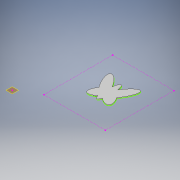
# Autodesk Inventor part: Butterfly
Saved by Autodesk Inventor 2019 (Build 230136000, 136)
## iProperties
Created: 2019-02-04
Part Number: Butterfly
Material: Generic
Document SubType Name: Modeling
Designer: mrhftc
Density: 1 g/cm^3
Appearance: Default
Author: mrhftc
Autodesk Inventor part; units mm, degrees
ref_plane "YZ Plane" through (0, 0, 0) normal (1, 0, 0) x (0, 1, 0)
ref_plane "XZ Plane" through (0, 0, 0) normal (0, 1, 0) x (-1, 0, 0)
ref_plane "XY Plane" through (0, 0, 0) normal (0, 0, 1) x (1, 0, 0)
ref_plane "Work Plane2" through (0, 2.54, 0) normal (0, 1, 0) x (1, 0, 0)
sketch "Sketch5" plane through (0, 2.54, 0) normal (0, 1, 0) x (1, 0, 0)
  ellipse E0 centre (201.451, 177.3473) end of major axis (229.2052, 221.1135) minor radius 16.0156 (208.013, 158.6416) -> (186.5008, 183.6371) ccw
  ellipse E1 centre (187.6899, 154.5313) end of major axis (215.633, 123.3862) minor radius 18.4642 (184.5561, 132.1117) -> (208.013, 158.6416) ccw
  ellipse E2 centre (176.9986, 162.7883) end of major axis (176.9986, 205.3655) minor radius 10.8982 (186.5008, 183.6371) -> (176.9986, 205.3655) ccw
  ellipse E3 centre (176.9986, 162.7883) end of major axis (176.9986, 205.3655) minor radius 10.8982 (176.9986, 120.211) -> (184.5561, 132.1117) ccw
  ellipse E4 centre (152.5463, 177.3473) end of major axis (124.7921, 221.1135) minor radius 16.0156 (167.4964, 183.6371) -> (145.9843, 158.6416) ccw
  ellipse E5 centre (166.3073, 154.5313) end of major axis (138.3642, 123.3862) minor radius 18.4642 (145.9843, 158.6416) -> (169.4411, 132.1117) ccw
  ellipse E6 centre (176.9986, 162.7883) end of major axis (176.9986, 205.3655) minor radius 10.8982 (176.9986, 205.3655) -> (167.4964, 183.6371) ccw
  ellipse E7 centre (176.9986, 162.7883) end of major axis (176.9986, 205.3655) minor radius 10.8982 (169.4411, 132.1117) -> (176.9986, 120.211) ccw
  ellipse E8 centre (166.3073, 154.5313) end of major axis (138.3642, 123.3862) minor radius 18.4642 (145.9843, 158.6416) -> (169.4411, 132.1117) ccw
  ellipse E9 centre (187.6899, 154.5313) end of major axis (215.633, 123.3862) minor radius 18.4642 (184.5561, 132.1117) -> (208.013, 158.6416) ccw
  point P0 (0, 0)
  constraints: 2 coincident, 40 other
ref_plane "Work Plane1" through (0, 2.54, 0) normal (0, 1, 0) x (1, 0, 0)
sketch "Sketch7" plane through (0, 2.54, 0) normal (0, 1, 0) x (1, 0, 0)
  ellipse E0 centre (152.5463, 177.3473) end of major axis (124.7921, 221.1135) minor radius 16.0156 (167.4964, 183.6371) -> (145.9843, 158.6416) ccw construction
  ellipse E1 centre (176.9986, 162.7883) end of major axis (176.9986, 205.3655) minor radius 10.8982 (186.5008, 183.6371) -> (167.4964, 183.6371) ccw construction
  ellipse E2 centre (201.451, 177.3473) end of major axis (229.2052, 221.1135) minor radius 16.0156 (208.013, 158.6416) -> (186.5008, 183.6371) ccw construction
  ellipse E3 centre (187.6899, 154.5313) end of major axis (215.633, 123.3862) minor radius 18.4642 (184.5561, 132.1117) -> (208.013, 158.6416) ccw construction
  ellipse E4 centre (176.9986, 162.7883) end of major axis (176.9986, 205.3655) minor radius 10.8982 (169.4411, 132.1117) -> (184.5561, 132.1117) ccw construction
  line L0 (69.0486, 42.1383) -> (284.9486, 42.1383) construction
  line L1 (284.9486, 42.1383) -> (284.9486, 283.4383) construction
  line L2 (284.9486, 283.4383) -> (69.0486, 283.4383) construction
  line L3 (69.0486, 283.4383) -> (69.0486, 42.1383) construction
  ellipse E5 centre (166.3073, 154.5313) end of major axis (138.3642, 123.3862) minor radius 19.3992 (185.7346, 188.2439) -> (189.2792, 188.024) ccw
  ellipse E6 centre (176.9986, 162.7883) end of major axis (176.9986, 205.3655) minor radius 10.8982
  ellipse E7 centre (152.5463, 177.3473) end of major axis (124.7921, 221.1135) minor radius 16.0156
  ellipse E8 centre (187.6899, 154.5313) end of major axis (215.633, 123.3862) minor radius 18.4642 (164.8018, 187.896) -> (168.2101, 187.9664) ccw
  ellipse E9 centre (187.6899, 154.5313) end of major axis (215.633, 123.3862) minor radius 18.4642 (184.5561, 132.1117) -> (208.013, 158.6416) ccw construction
  ellipse E10 centre (201.451, 177.3473) end of major axis (229.2052, 221.1135) minor radius 16.0156
  ellipse E11 centre (176.9986, 162.7883) end of major axis (176.9986, 205.3655) minor radius 10.8982
  ellipse E12 centre (152.5463, 177.3473) end of major axis (124.7921, 221.1135) minor radius 16.0156 (145.4208, 159.4026) -> (163.4994, 189.8573) ccw
  ellipse E13 centre (201.451, 177.3473) end of major axis (229.2052, 221.1135) minor radius 16.0156
  point P0 (0, 0)
  constraints: 8 coincident, 33 other
extrude "Extrusion7" add sketch "Sketch5" along normal blind 2.54
body "Solid2"
